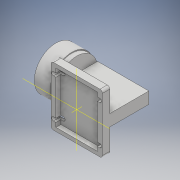
# Autodesk Inventor part: boquilla_capnografo_V1
Saved by Autodesk Inventor 2018 (Build 220112000, 112)
## iProperties
Created: 2020-04-02
Part Number: boquilla_capnografo_V1
Material: Generic
Document SubType Name: Modeling
Designer: antonio
Density: 1 g/cm^3
Appearance: Default
Author: antonio
Autodesk Inventor part; units mm, degrees
ref_plane "YZ Plane" through (0, 0, 0) normal (1, 0, 0) x (0, 1, 0)
ref_plane "XZ Plane" through (0, 0, 0) normal (0, 1, 0) x (-1, 0, 0)
ref_plane "XY Plane" through (0, 0, 0) normal (0, 0, 1) x (1, 0, 0)
sketch "Sketch1" plane through (0, 0, 0) normal (0, 1, 0) x (-1, 0, 0)
  line L0 (29.9799, 0) -> (-29.9799, 0) projected
  line L1 (0, -34.1799) -> (0, 34.1799) projected
  line L2 (19, 24) -> (-19, 24)
  line L3 (-21, 22) -> (-21, -22)
  line L4 (-19, -24) -> (19, -24)
  line L5 (21, -22) -> (21, 22)
  arc A0 (21, 22) -> (19, 24) centre (19, 22) ccw
  arc A1 (19, -24) -> (21, -22) centre (19, -22) ccw
  arc A2 (-21, -22) -> (-19, -24) centre (-19, -22) ccw
  arc A3 (-19, 24) -> (-21, 22) centre (-19, 22) ccw
  point P0 (0, 0)
  point P1 (21, 24)
  point P2 (-21, -24)
  point P3 (-21, 24)
  point P4 (21, -24)
  dimension "d0" = 42
  dimension "d1" = 48
  dimension "d4" = 2
  constraints: 8 end point, 8 point on circle, 8 point on line, 8 tangent, 4 centre point, 3 equal radius, 2 parallel, 1 horizontal, 1 perpendicular, 2 other
  measures "d0" distance of point (21, -24) point (-21, -24)
  measures "d1" distance of point (-21, -24) point (-21, 24)
  measures "d4" radius of A0
extrude "Extrusion1" add sketch "Sketch1" along normal blind 6
sketch "Sketch2" plane through (0, 0, 0) normal (0, -1, 0) x (1, 0, 0)
  line L0 (-29.4, 0) -> (29.4, 0) projected
  line L1 (0, -33.6) -> (0, 33.6) projected
  line L2 (17, 21) -> (-17, 21)
  line L3 (-17, 21) -> (-17, -21)
  line L4 (-17, -21) -> (17, -21)
  line L5 (17, -21) -> (17, 21)
  point P0 (0, 0)
  dimension "d5" = 34
  dimension "d6" = 42
  constraints: 8 end point, 2 parallel, 1 horizontal, 1 perpendicular, 2 other
  measures "d5" distance of L4.end L3.end
  measures "d6" distance of L3.end L2.end
extrude "Extrusion2" cut sketch "Sketch2" against normal blind 4
sketch "Sketch3" plane through (0, 6, 0) normal (0, 1, 0) x (1, 0, 0)
  line L0 (-29.4, 0) -> (29.4, 0) projected
  line L1 (0, 33.6) -> (0, -33.6) projected
  line L2 (19, 16) -> (15, 16) construction
  line L3 (17, -21) -> (17, 21) projected
  line L4 (19, 17.5) -> (15, 17.5)
  line L5 (15, 14.5) -> (19, 14.5)
  arc A0 (19, 14.5) -> (19, 17.5) centre (19, 16) ccw
  arc A1 (15, 17.5) -> (15, 14.5) centre (15, 16) ccw
  line L6 (19, 16) -> (23, 16) construction
  line L7 (21, -22) -> (21, 22) projected
  line L8 (19, 24) -> (-19, 24) projected
  point P0 (0, 0)
  point P1 (17, 16)
  dimension "d9" = 4
  dimension "d10" = 180
  dimension "d11" = 3
  dimension "d12" = 4
  dimension "d13" = 8
  constraints: 10 end point, 4 point on circle, 4 tangent, 2 centre point, 1 collinear, 1 horizontal, 1 midpoint, 1 parallel, 1 perpendicular
  measures "d9" distance of L2.start L2.end
  measures "d10" angle of L2 L6
  measures "d11" diameter of A1
  measures "d12" distance from line of L7 point (17, 16)
  measures "d13" distance from line of L8 point (17, 16)
extrude "Extrusion3" cut sketch "Sketch3" against normal through all
mirror "Mirror1" about plane through (0, 0, 0) normal (0, 0, 1) of "Extrusion3"
mirror "Mirror2" about plane through (0, 0, 0) normal (1, 0, 0) of "Extrusion3", "Mirror1"
sketch "Sketch4" plane through (0, 6, 0) normal (0, 1, 0) x (1, 0, 0)
  line L0 (21, 4.75) -> (-21, 4.75)
  line L1 (-21, 4.75) -> (-21, -4.75)
  line L2 (-21, -4.75) -> (21, -4.75)
  line L3 (21, -4.75) -> (21, 4.75)
  line L4 (21, -22) -> (21, 22) projected
  line L5 (-21, 22) -> (-21, -22) projected
  line L6 (-29.4, 0) -> (29.4, 0) projected
  point P0 (0, 0)
  dimension "d16" = 9.5
  constraints: 8 end point, 2 collinear, 2 parallel, 1 horizontal, 1 perpendicular, 1 other
  measures "d16" distance between parallel lines of L0 L2
extrude "Extrusion4" add sketch "Sketch4" along normal blind 32
sketch "Sketch5" plane through (-21, 0, -22) normal (-1, 0, 0) x (0, 0, 1)
  circle A0 centre (22, 21) radius 17
  line L0 (17.25, 38) -> (26.75, 38) projected
  line L1 (22, -7.6) -> (22, 45.6) projected
  point P0 (22, 0)
  dimension "d19" = 34
  constraints: 1 centre point, 1 point on line, 1 tangent
  measures "d19" diameter of A0
extrude "Extrusion5" add sketch "Sketch5" along normal blind 4
sketch "Sketch6" plane through (-25, 21, 0) normal (-1, 0, 0) x (0, 0, 1)
  circle A0 centre (0, 0) radius 17 projected
  circle A1 centre (0, 0) radius 17.7
  point P0 (0, -21)
  dimension "d22" = 35.4
  constraints: 1 centre point, 1 coincident
  measures "d22" diameter of A1
extrude "Extrusion6" add sketch "Sketch6" along normal blind 13 contours A0 | A1
sketch "Sketch7" plane through (-38, 21, 0) normal (-1, 0, 0) x (0, 0, 1)
  circle A0 centre (0, 0) radius 17.7 projected
  circle A1 centre (0, 0) radius 15
  point P0 (0, -21)
  dimension "d25" = 30
  constraints: 1 centre point, 1 coincident
  measures "d25" diameter of A1
extrude "Extrusion7" cut sketch "Sketch7" against normal blind 12 contours A1
sketch "Sketch8" plane through (-26, 21, 0) normal (-1, 0, 0) x (0, 0, 1)
  line L0 (-3.75, 14.5237) -> (3.75, 14.5237)
  line L1 (3.75, 14.5237) -> (3.75, -13.9763)
  line L2 (3.75, -13.9763) -> (-3.75, -13.9763)
  line L3 (-3.75, -13.9763) -> (-3.75, 14.5237)
  circle A0 centre (0, 0) radius 15 projected
  line L4 (0, -28.74) -> (0, 25.44) projected
  point P0 (0, -21)
  dimension "d28" = 7.5
  dimension "d29" = 28.5
  constraints: 8 end point, 2 parallel, 1 horizontal, 1 perpendicular, 3 other
  measures "d28" distance of L1.end L2.end
  measures "d29" distance of L0.end L1.end
extrude "Extrusion8" cut sketch "Sketch8" against normal blind 45 contours L0 L4 L2 L3 | L0 L1 L2 L4
body "Solid1"
